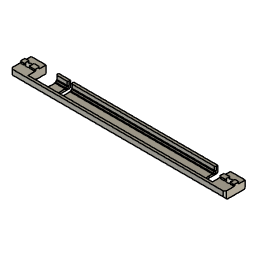
rear_gantry_wire_cover (Autodesk Fusion 360 design; units mm, degrees)
Autodesk Fusion 360 part; units mm, degrees
sketch "Sketch1" plane through (0, 0, 0) normal (1, 0, 0) x (0, 1, 0)
  line L0 (0, 0) -> (13, 0)
  line L1 (13, 0) -> (13, 4.6)
  line L2 (13, 4.6) -> (11.4, 4.6)
  line L3 (11.4, 4.6) -> (11.4, 1)
  line L4 (11.4, 1) -> (1.6, 1)
  line L5 (1.6, 1) -> (1.6, 5.2)
  line L6 (1.6, 5.2) -> (0, 5.2)
  line L7 (0, 5.2) -> (0, 0)
  dimension "d1" = 5.2
  dimension "d2" = 1.6
  dimension "d3" = 1
  dimension "d4" = 4.6
  dimension "d5" = 13
  constraint coincident L0.start L7.end
  constraint horizontal L0
  constraint perpendicular L0 L1
  constraint perpendicular L1 L2
  constraint perpendicular L2 L3
  constraint perpendicular L3 L4
  constraint perpendicular L4 L5
  constraint perpendicular L3 L6
  constraint perpendicular L0 L7
  constraint equal L2 L6
  measures "d1" distance of L6.end L0.start
  measures "d2" distance of L5.end L6.end
  measures "d3" distance of L0 L4
  measures "d4" distance of L0.end L1.end
  measures "d5" distance of L0.start L0.end
extrude "Extrude1" add sketch "Sketch1" along normal blind 136
ref_plane "WorkPlane1" through (68, 0.8, 5.2) normal (0, 0, 1) x (0, -1, 0)
sketch "Sketch2" plane through (0, 0, 5.2) normal (0, 0, 1) x (1, 0, 0)
  line L0 (0, 0) -> (0, 13)
  line L1 (0, 13) -> (136, 13)
  line L2 (136, 13) -> (136, 0)
  line L3 (136, 0) -> (0, 0)
  line L4 (0, 7.5) -> (136, 7.5) construction
  circle A0 centre (131.8, 7.5) radius 1.7
  circle A1 centre (131.8, 7.5) radius 4.2 construction
  line L5 (126.6, 13) -> (126.6, 7.5)
  line L6 (118.6, 13) -> (118.6, 7.5)
  arc A2 (118.6, 7.5) -> (126.6, 7.5) centre (122.6, 7.5) ccw
  line L7 (68, 13) -> (68, 0) construction
  line L8 (126.6, 7.5) -> (126.6, 0)
  circle A3 centre (4.2, 7.5) radius 1.7
  line L9 (9.4, 7.5) -> (9.4, 0)
  line L10 (9.4, 13) -> (9.4, 7.5)
  arc A4 (9.4, 7.5) -> (17.4, 7.5) centre (13.4, 7.5) ccw
  line L11 (17.4, 13) -> (17.4, 7.5)
  line L12 (27, 13) -> (27, 6)
  line L13 (25, 13) -> (25, 6)
  arc A5 (25, 6) -> (27, 6) centre (26, 6) ccw
  line L14 (0, 9) -> (9.4, 9)
  line L15 (0, 6) -> (9.4, 6)
  line L16 (136, 9) -> (126.6, 9)
  line L17 (136, 6) -> (126.6, 6)
  dimension "d9" = 3.4
  dimension "d10" = 8.4
  dimension "d11" = 7.5
  dimension "d12" = 1
  dimension "d13" = 4
  dimension "d14" = 110
  dimension "d15" = 1
  dimension "d16" = 1.5
  dimension "d29" = 3
  constraint coincident L0 L4.start
  constraint coincident L2 L4.end
  constraint perpendicular L2 L4
  constraint coincident L4 A0.centre
  constraint concentric A0 A1
  constraint tangent L2 A1
  constraint coincident L1 L5.start
  constraint perpendicular L4 L5
  constraint coincident L1 L6.start
  constraint perpendicular L4 L6
  constraint tangent L6 A2
  constraint tangent L5 A2
  constraint coincident L4 A2.centre
  constraint midpoint L1 L7.start
  constraint midpoint L3 L7.end
  constraint coincident L3 L8.end
  constraint tangent A2 L8
  constraint symmetric A0 L7 A3
  constraint symmetric L5.start L7 L10.start
  constraint symmetric L5.end L7 L9.start
  constraint symmetric L6.start L7 L11.start
  constraint symmetric L6.end L7 A4.end
  constraint symmetric A2 L7 A4
  constraint symmetric L7 L8.end L9.end
  constraint coincident L1 L12.start
  constraint perpendicular L4 L12
  constraint coincident L1 L13.start
  constraint perpendicular L4 L13
  constraint tangent L13 A5
  constraint tangent L12 A5
  constraint coincident L0 L14.start
  constraint coincident L10 L14.end
  constraint perpendicular L10 L14
  constraint symmetric L4 L14.start L15.start
  constraint symmetric L4 L14.end L15.end
  constraint symmetric L7 L14.start L16.start
  constraint symmetric L7 L14.end L16.end
  constraint symmetric L7 L15.start L17.start
  constraint symmetric L7 L15.end L17.end
  measures "d9" diameter of A0
  measures "d10" diameter of A1
  measures "d11" distance of L3 L4
  measures "d12" distance of A1 L5
  measures "d13" radius of A2
  measures "d14" distance of L2 A5.centre
  measures "d15" radius of A5
  measures "d16" distance of L4 A5.centre
  measures "d29" distance of L14 L15
extrude "Extrude2" add sketch "Sketch2" against normal up to surface (4.2 mm away) contours L0 L3 A3 L9 L15 | L0 A3 L14 L15 | L0 L1 A3 L10 L14 | L2 L3 A0 L8 L17 | A3 L9 L10 L14 L15 | A0 L5 L8 L16 L17 | L2 A0 L16 L17 | L1 L2 A0 L5 L16
extrude "Extrude8" cut 2 faces at (3.6895, 7.7459, 1) (132.0833, 6.5175, 1) along direction (0, 0, 1) up to surface end surface through (0, 0, 0) normal (0, 0, -1) offset 0
extrude "Extrude3" cut sketch "Sketch2" against normal up to surface (5.2 mm away) contours L1 L10 A4 L11 | L1 L5 L6 A2 | L1 L12 L13 A5
extrude "Extrude4" add sketch "Sketch2" along normal blind 1 contours L0 A3 L14 L15 | A3 L9 L10 L14 L15 | A0 L5 L8 L16 L17 | L2 A0 L16 L17
fillet "Fillet2" radius 0.4 16 edges at (131, 9, 5.7) (132.6, 9, 5.7) (131, 6, 5.7) (126.6, 6, 5.7) (126.6, 9, 5.7) (136, 9, 5.7) (132.6, 6, 5.7) (136, 6, 5.7) (0, 6, 5.7) (0, 9, 5.7) (3.4, 9, 5.7) (3.4, 6, 5.7) (5, 9, 5.7) (5, 6, 5.7) (9.4, 6, 5.7) (9.4, 9, 5.7)
chamfer "Chamfer1" distance 2 angle 45 1 edges at (68, 0, 0)
chamfer "Chamfer2" distance 1 angle 45 2 edges at (0, 0, 3.6) (136, 0, 3.6)
chamfer "Chamfer3" distance 1 angle 45 5 edges at (72.8, 11.4, 1) (21.2, 11.4, 1) (131.3, 13, 0) (72.8, 13, 0) (21.2, 13, 0)
chamfer "Chamfer4" distance 0.4 angle 45 9 edges at (122.6, 3.5, 0) (118.6, 9.75, 0) (126.6, 9.75, 0) (26, 5, 0) (25, 9, 0) (27, 9, 0) (13.4, 3.5, 0) (9.4, 10.25, 0) (17.4, 9.75, 0)
chamfer "Chamfer5" distance 1.4 angle 45 1 edges at (68, 1.6, 1)
fillet "Fillet1" radius 0.6 19 edges at (122.6, 3.5, 1) (118.6, 8.95, 1) (27, 8.2, 1) (26, 5, 1) (25, 8.2, 1) (17.4, 8.95, 1) (13.4, 3.5, 1) (17.4, 10.9, 1.5) (17.4, 11.4, 3.3) (21.2, 10.4, 1) (21.2, 11.4, 2) (72.8, 11.4, 2) (27, 10.9, 1.5) (25, 10.9, 1.5) (25, 11.4, 3.3) (27, 11.4, 3.3) (72.8, 10.4, 1) (118.6, 10.9, 1.5) (118.6, 11.4, 3.3)
sketch "Sketch3" plane through (0, 0, 0) normal (0, 0, -1) x (1, 0, 0)
  line L0 (17.8, -7.5) -> (17.8, -12)
  line L1 (17.8, -12) -> (24.6, -12)
  line L2 (24.6, -12) -> (24.6, -6)
  arc A0 (27.4, -6) -> (24.6, -6) centre (26, -6) ccw
  line L3 (27.4, -6) -> (27.4, -12)
  line L4 (27.4, -12) -> (118.2, -12)
  line L5 (118.2, -12) -> (118.2, -7.5)
  arc A1 (127, -7.5) -> (118.2, -7.5) centre (122.6, -7.5) ccw
  line L6 (127, -7.5) -> (127, -12)
  line L7 (127, -12) -> (136, -12)
  line L8 (136, -12) -> (136, -2)
  line L9 (136, -2) -> (0, -2)
  line L10 (0, -2) -> (0, -13)
  line L11 (0, -13) -> (9, -13)
  line L12 (9, -13) -> (9, -7.5)
  arc A2 (17.8, -7.5) -> (9, -7.5) centre (13.4, -7.5) ccw
  circle A3 centre (4.2, -7.5) radius 1.7
  circle A4 centre (131.8, -7.5) radius 1.7
  circle A5 centre (4.2, -7.5) radius 3
  line L13 (5.9, -5.0282) -> (5.9, -9.9718)
  line L14 (2.5, -9.9718) -> (2.5, -5.0282)
  line L15 (5.9, -9.2) -> (2.5, -9.2)
  line L16 (5.9, -5.8) -> (2.5, -5.8)
  circle A6 centre (4.2, -7.5) radius 1.7
  line L17 (68, -2) -> (68, -12) construction
  circle A7 centre (131.8, -7.5) radius 3
  line L18 (130.1, -9.2) -> (133.5, -9.2)
  line L19 (130.1, -5.0282) -> (130.1, -9.9718)
  line L20 (133.5, -9.9718) -> (133.5, -5.0282)
  line L21 (130.1, -5.8) -> (133.5, -5.8)
  dimension "d34" = 6
  constraint concentric A3 A5
  constraint coincident A5 L13.start
  constraint coincident A5 L13.end
  constraint vertical L13
  constraint coincident A5 L14.start
  constraint coincident L13 L15.start
  constraint coincident L14 L15.end
  constraint perpendicular L14 L15
  constraint coincident L13 L16.start
  constraint coincident L14 L16.end
  constraint perpendicular L14 L16
  constraint coincident A5 L14.end
  constraint parallel L13 L14
  constraint tangent A3 L13
  constraint tangent A3 L15
  constraint tangent L14 A6
  constraint tangent A3 L16
  constraint midpoint L9 L17.start
  constraint coincident L4 L17.end
  constraint perpendicular L4 L17
  constraint symmetric A5 L17 A7
  constraint symmetric L13.start L17 L19.start
  constraint symmetric L13.end L17 L19.end
  constraint symmetric L14.start L17 L20.start
  constraint symmetric L14.end L17 L20.end
  constraint symmetric L15.start L17 L18.start
  constraint symmetric L15.end L17 L18.end
  constraint symmetric L16.start L17 L21.start
  constraint symmetric L16.end L17 L21.end
  measures "d34" diameter of A5
extrude "Extrude5" cut sketch "Sketch3" against normal blind 2.4 contours A3 L13 L15 A6 | A3 L13 L16 A6 | A3 L14 L16 A6 | A3 L14 L15 A6 | A4 L18 L20 | A4 L20 L21 | A4 L19 L21 | A4 L18 L19
extrude "Extrude6" cut sketch "Sketch3" against normal blind 2.2 contours A5 L13 L14 L16 | A5 L13 L14 L15 | A7 L19 L20 L21 | A7 L18 L19 L20
extrude "Extrude7" cut sketch "Sketch3" against normal blind 2 contours A5 L13 | A5 L14 | A7 L20 | A7 L19
chamfer "Chamfer6" distance 0.4 angle 45 5 edges at (0, 7.5, 0) (4.5, 13, 0) (136, 7, 0) (129.003, 6.4152, 0) (1.403, 6.4152, 0)
